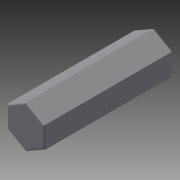
# Autodesk Inventor part: 000107-1
Saved by Autodesk Inventor 2015 (Build 190159000, 159)
## iProperties
Created: 2015-05-11
Part Number: 000107-1
Material: Generic
Document SubType Name: Modeling
Designer: Wesley
Density: 1 g/cm^3
Appearance: Default
Author: Wesley
Autodesk Inventor part; units mm, degrees
ref_plane "YZ Plane" through (0, 0, 0) normal (1, 0, 0) x (0, 1, 0)
ref_plane "XZ Plane" through (0, 0, 0) normal (0, 1, 0) x (-1, 0, 0)
ref_plane "XY Plane" through (0, 0, 0) normal (0, 0, 1) x (1, 0, 0)
sketch "Sketch1" plane through (0, 0, 0) normal (0, 0, 1) x (1, 0, 0)
  line L0 (0, 3.175) -> (2.7496, 1.5875)
  line L1 (2.7496, 1.5875) -> (2.7496, -1.5875)
  line L2 (2.7496, -1.5875) -> (0, -3.175)
  line L3 (0, -3.175) -> (-2.7496, -1.5875)
  line L4 (-2.7496, -1.5875) -> (-2.7496, 1.5875)
  line L5 (-2.7496, 1.5875) -> (0, 3.175)
  point P0 (0, 0)
  point P1 (0, 0)
  dimension "d0" = 6.35
  dimension "d1" = 3.175
  dimension "d2" = 2.7496
  constraints: 12 end point, 1 coincident, 13 other
  measures "d0" distance of L2.end L0.start
  measures "d1" distance of L0.end L1.end
  measures "d2" horizontal distance of L0.start L0.end
extrude "Extrusion1" add sketch "Sketch1" along normal blind 19.05
fillet "Fillet1" radius 0.254 12 edges at (-1.3748, 2.3812, 19.05) (-2.7496, 0, 19.05) (-1.3748, -2.3813, 19.05) (1.3748, -2.3813, 19.05) (2.7496, 0, 19.05) (1.3748, 2.3812, 19.05) (-1.3748, 2.3812, 0) (1.3748, 2.3812, 0) (2.7496, 0, 0) (1.3748, -2.3813, 0) (-1.3748, -2.3813, 0) (-2.7496, 0, 0)
body "Solid1"
